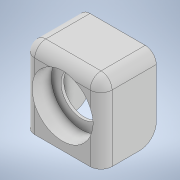
# Autodesk Inventor part: mocowanie lozyska 10-2
Saved by Autodesk Inventor 2021 (Build 250183000, 183)
## iProperties
Created: 2021-11-06
Part Number: mocowanie lozyska 10-2
Material: Generic
Document SubType Name: Modeling
Designer: Łukasz
Density: 1 g/cm^3
Appearance: Default
Author: Łukasz
Autodesk Inventor part; units mm, degrees
ref_plane "YZ Plane" through (0, 0, 0) normal (1, 0, 0) x (0, 1, 0)
ref_plane "XZ Plane" through (0, 0, 0) normal (0, 1, 0) x (-1, 0, 0)
ref_plane "XY Plane" through (0, 0, 0) normal (0, 0, 1) x (1, 0, 0)
sketch "Sketch1" plane through (0, 0, 0) normal (0, 0, 1) x (1, 0, 0)
  circle A0 centre (0, 0) radius 7.5
  line L0 (-10, 10) -> (10, 10)
  line L1 (10, 10) -> (10, -10)
  line L2 (10, -10) -> (-10, -10)
  line L3 (-10, -10) -> (-10, 10)
  line L4 (-10, -10) -> (-14, -10)
  line L5 (-14, -10) -> (-14, 10)
  line L6 (-14, 10) -> (-10, 10)
  line L7 (-10, 10) -> (-10, -10)
  line L8 (10, -10) -> (14, -10)
  line L9 (14, -10) -> (14, 10)
  line L10 (14, 10) -> (10, 10)
  line L11 (10, 10) -> (10, -10)
  line L12 (14, 10) -> (-14, 10)
  line L13 (-14, 10) -> (-14, 14)
  line L14 (-14, 14) -> (14, 14)
  line L15 (14, 14) -> (14, 10)
  line L16 (14, -10) -> (-14, -10)
  line L17 (-14, -10) -> (-14, -14)
  line L18 (-14, -14) -> (14, -14)
  line L19 (14, -14) -> (14, -10)
  dimension "d0" = 15
  dimension "d1" = 20
  dimension "d2" = 20
  dimension "d3" = 4
  dimension "d4" = 4
  dimension "d5" = 4
  dimension "d9" = 4
  constraints: 40 end point, 10 parallel, 5 horizontal, 5 perpendicular, 3 point on line, 1 centre point, 1 coincident
  measures "d0" diameter of A0
  measures "d1" distance of L1.end L2.end
  measures "d2" distance of L0.end L1.end
  measures "d3" distance of L5.end L6.end
  measures "d4" distance of L10.end L9.end
  measures "d5" distance of L12.end L13.end
  measures "d9" distance of L17.end L16.end
extrude "Extrusion1" add sketch "Sketch1" along normal blind 1
sketch "Sketch2" plane through (0, 0, 1) normal (0, 0, 1) x (1, 0, 0)
  circle A0 centre (0, 0) radius 7.5 projected
  circle A1 centre (0, 0) radius 11
  line L0 (14, 14) -> (-14, 14) projected
  circle A2 centre (0, 0) radius 7.5 projected
  line L1 (-14, 14) -> (-14, -14) projected
  line L2 (-14, -14) -> (14, -14) projected
  line L3 (14, -14) -> (14, 14) projected
  dimension "d8" = 22
  constraints: 1 centre point, 1 coincident
  measures "d8" diameter of A1
extrude "Extrusion2" add sketch "Sketch2" along normal blind 7 contours L3 L2 L1 L0
sketch "Sketch3" plane through (0, 0, 0) normal (0, 0, -1) x (-1, 0, 0)
  line L0 (14, 14) -> (14, -14) projected
  line L1 (-14, 14) -> (14, 14) projected
  line L2 (-14, -14) -> (-14, 14) projected
  line L3 (14, -14) -> (-14, -14) projected
  circle A0 centre (0, 0) radius 7.5 projected
  line L4 (10, 10) -> (10, -10)
  line L5 (10, -10) -> (-10, -10)
  line L6 (-10, -10) -> (-10, 10)
  line L7 (-10, 10) -> (10, 10)
  line L8 (-10, -10) -> (-10, -14)
  line L9 (10, -10) -> (10, -14)
  line L10 (14, -14) -> (-14, -14) projected
  dimension "d12" = 4
  constraints: 12 end point, 2 point on line, 1 parallel, 1 perpendicular, 3 other
  measures "d12" distance between parallel lines of L1 L7
extrude "Extrusion3" add sketch "Sketch3" along normal blind 12 contours L0 L3 L9 L4 L7 L6 L8 L2 L1
fillet "Fillet1" radius 6 2 edges at (-12, -14, -12) (12, -14, -12)
fillet "Fillet2" radius 4 5 edges at (-14, 14, -2) (0, 14, 8) (14, 14, -2) (-14, 0, 8) (14, 0, 8)
body "Solid1"
